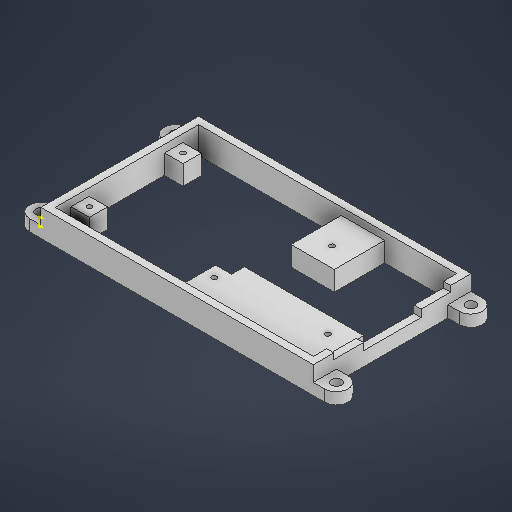
# Autodesk Inventor part: lock2
Saved by Autodesk Inventor 2026 (Build 300175050, 175E)
## iProperties
Created: 2025-07-25
Part Number: lock2
Material: Generic
Document SubType Name: Modeling
Designer: User
Density: 1 g/cm^3
Appearance: Default
Author: User
Autodesk Inventor part; units mm, degrees
ref_plane "YZ Plane" through (0, 0, 0) normal (1, 0, 0) x (0, 1, 0)
ref_plane "XZ Plane" through (0, 0, 0) normal (0, 1, 0) x (-1, 0, 0)
ref_plane "XY Plane" through (0, 0, 0) normal (0, 0, 1) x (1, 0, 0)
sketch "Sketch1" plane through (0, 0, 0) normal (0, 1, 0) x (-1, 0, 0)
  line L0 (0, 0) -> (-94.5, 0)
  line L1 (-94.5, 0) -> (-94.5, -54.7)
  line L2 (-94.5, -54.7) -> (0, -54.7)
  line L3 (0, -54.7) -> (0, 0)
  dimension "d0" = 94.5
  dimension "d1" = 54.7
  constraints: 8 end point, 2 parallel, 1 horizontal, 1 perpendicular
  measures "d0" distance of L2.end L1.end
  measures "d1" distance of L1.end L0.end
extrude "Extrusion1" add sketch "Sketch1" along normal blind 9.3
sketch "Sketch2" plane through (0, 9.3, 0) normal (0, 1, 0) x (1, 0, 0)
  line L0 (2.5, 2.5) -> (92, 2.5)
  line L1 (92, 2.5) -> (92, 52.2)
  line L2 (92, 52.2) -> (2.5, 52.2)
  line L3 (2.5, 52.2) -> (2.5, 2.5)
  line L4 (0, 0) -> (94.5, 0) projected
  line L5 (0, 54.7) -> (0, 0) projected
  dimension "d4" = 89.5
  dimension "d5" = 49.7
  dimension "d6" = 2.5
  dimension "d7" = 2.5
  constraints: 8 end point, 2 parallel, 1 horizontal, 1 perpendicular
  measures "d4" distance of L2.end L1.end
  measures "d5" distance of L1.end L0.end
  measures "d6" distance between parallel lines of L4 L0
  measures "d7" distance between parallel lines of L5 L3
extrude "Extrusion2" cut sketch "Sketch2" against normal blind 2.5
sketch "Sketch3" plane through (0, 6.8, 0) normal (0, 1, 0) x (1, 0, 0)
  point P0 (0, 0)
sketch "Sketch4" plane through (0, 6.8, 0) normal (0, 1, 0) x (1, 0, 0)
  line L0 (2.6094, 40.3) -> (9.0094, 40.3)
  line L1 (9.0094, 40.3) -> (9.0094, 46.6)
  line L2 (9.0094, 46.6) -> (2.6094, 46.6)
  line L3 (2.6094, 46.6) -> (2.6094, 40.3)
  line L4 (2.5, 52.2) -> (92, 52.2) projected
  line L5 (2.5, 2.5) -> (2.5, 52.2) projected
  line L6 (2.5, 7.905) -> (8.9, 7.905)
  line L7 (8.9, 7.905) -> (8.9, 14.205)
  line L8 (8.9, 14.205) -> (2.5, 14.205)
  line L9 (2.5, 14.205) -> (2.5, 7.905)
  line L10 (92, 2.5) -> (2.5, 2.5) projected
  line L11 (45.1276, 2.5) -> (95.6526, 2.5)
  line L12 (95.6526, 2.5) -> (95.6526, 19.973)
  line L13 (95.6526, 19.973) -> (45.1276, 19.973)
  line L14 (45.1276, 19.973) -> (45.1276, 2.5)
  line L15 (52.018, 52.2) -> (67.018, 52.2)
  line L16 (67.018, 52.2) -> (67.018, 34.727)
  line L17 (67.018, 34.727) -> (52.018, 34.727)
  line L18 (52.018, 34.727) -> (52.018, 52.2)
  line L19 (92, 52.2) -> (92, 2.5) projected
  point P0 (0, 0)
  point P1 (5.8094, 46.6)
  point P2 (5.7, 7.905)
  point P3 (67.018, 43.4635)
  point P4 (92, 19.973)
  point P5 (2.5, 14.205)
  dimension "d10" = 6.4
  dimension "d11" = 6.3
  dimension "d12" = 5.6
  dimension "d13" = 6.4
  dimension "d14" = 6.3
  dimension "d15" = 5.405
  dimension "d16" = 50.525
  dimension "d17" = 17.473
  dimension "d18" = 15
  dimension "d19" = 17.473
  dimension "d20" = 24.982
  constraints: 32 end point, 8 parallel, 4 horizontal, 4 perpendicular, 3 midpoint, 3 point on line
  measures "d10" distance of L2.end L1.end
  measures "d11" distance of L1.end L0.end
  measures "d12" distance from line of L4 point (5.809, 46.6)
  measures "d13" distance of L8.end L7.end
  measures "d14" distance of L7.end L6.end
  measures "d15" distance from line of point (5.7, 7.905) L10
  measures "d16" distance of L13.end L12.end
  measures "d17" distance of L12.end L11.end
  measures "d18" distance of L16.end L17.end
  measures "d19" distance of L15.end L16.end
  measures "d20" distance from line of L19 point (67.018, 43.464)
extrude "Extrusion3" cut sketch "Sketch4" against normal blind 10 contours L4 L18 L17 L16 L19 L13 L14 L10 L5 L6 L7 L8
sketch "Sketch5" plane through (0, 6.8, 0) normal (0, 1, 0) x (1, 0, 0)
  line L0 (45.1276, 2.5) -> (45.1276, 19.973) projected
  line L1 (45.1276, 19.973) -> (50.6276, 19.973)
  line L2 (50.6276, 19.973) -> (50.6276, 15.473)
  line L3 (50.6276, 15.473) -> (45.1276, 15.473)
  line L4 (45.1276, 15.473) -> (45.1276, 19.973)
  point P0 (0, 0)
  dimension "d23" = 5.5
  dimension "d24" = 4.5
  constraints: 8 end point, 2 parallel, 1 horizontal, 1 perpendicular
  measures "d23" distance of L2.end L3.end
  measures "d24" distance of L1.end L2.end
extrude "Extrusion4" cut sketch "Sketch5" against normal blind 10
sketch "Sketch6" plane through (0, 9.3, 0) normal (0, 1, 0) x (1, 0, 0)
  line L0 (92, 19.973) -> (92, 2.5) projected
  line L1 (94.5, 0) -> (94.5, 54.7) projected
  line L2 (92, 7.1) -> (94.5, 7.1)
  line L3 (94.5, 7.1) -> (94.5, 47.6)
  line L4 (94.5, 47.6) -> (92, 47.6)
  line L5 (92, 47.6) -> (92, 7.1)
  line L6 (94.5, 54.7) -> (0, 54.7) projected
  point P0 (0, 0)
  point P1 (93.25, 47.6)
  dimension "d27" = 40.5
  dimension "d28" = 7.1
  constraints: 8 end point, 2 parallel, 2 point on line, 1 horizontal, 1 midpoint, 1 perpendicular
  measures "d27" distance of L3.end L2.end
  measures "d28" distance from line of L6 point (93.25, 47.6)
extrude "Extrusion5" cut sketch "Sketch6" against normal blind 2
sketch "Sketch7" plane through (0, 7.3, 0) normal (0, 1, 0) x (1, 0, 0)
  line L0 (92, 19.973) -> (92, 2.5) projected
  line L1 (94.5, 0) -> (94.5, 54.7) projected
  line L2 (92, 17.35) -> (94.5, 17.35)
  line L3 (94.5, 17.35) -> (94.5, 37.35)
  line L4 (94.5, 37.35) -> (92, 37.35)
  line L5 (92, 37.35) -> (92, 17.35)
  line L6 (92, 47.6) -> (94.5, 47.6) projected
  point P0 (0, 0)
  point P1 (93.25, 47.6)
  point P2 (93.25, 37.35)
  dimension "d31" = 20
  dimension "d32" = 10.25
  constraints: 8 end point, 2 midpoint, 2 parallel, 2 point on line, 1 horizontal, 1 perpendicular
  measures "d31" distance of L3.end L2.end
  measures "d32" distance of point (93.25, 47.6) point (93.25, 37.35)
extrude "Extrusion6" cut sketch "Sketch7" against normal blind 2.5
sketch "Sketch8" plane through (0, 0, -54.7) normal (-1, 0, 0) x (0, 0, 1)
  line L0 (54.7, 0) -> (46.7, 0)
  line L1 (46.7, 0) -> (46.7, 4)
  line L2 (46.7, 4) -> (54.7, 4)
  line L3 (54.7, 4) -> (54.7, 0)
  line L4 (0, 0) -> (0, 9.3) projected
  line L5 (0, 0) -> (8, 0)
  line L6 (8, 0) -> (8, 4)
  line L7 (8, 4) -> (0, 4)
  line L8 (0, 4) -> (0, 0)
  point P0 (0, 4)
  point P1 (4, 0)
  point P2 (4, 4)
  dimension "d35" = 8
  dimension "d36" = 4
  dimension "d37" = 8
  dimension "d47" = 4
  constraints: 16 end point, 4 parallel, 2 horizontal, 2 midpoint, 2 perpendicular, 1 point on line
  measures "d35" distance of L1.end L2.end
  measures "d36" distance of L0.end L1.end
  measures "d37" distance of L7.end L6.end
  measures "d47" distance of point (4, 0) point (4, 4)
extrude "Extrusion7" add sketch "Sketch8" along normal blind 8
sketch "Sketch9" plane through (94.5, 0, 0) normal (1, 0, 0) x (0, 0, -1)
  line L0 (0, 0) -> (8, 0)
  line L1 (8, 0) -> (8, 4)
  line L2 (8, 4) -> (0, 4)
  line L3 (0, 4) -> (0, 0)
  line L4 (54.6278, 0) -> (46.6278, 0)
  line L5 (46.6278, 0) -> (46.6278, 4)
  line L6 (46.6278, 4) -> (54.6278, 4)
  line L7 (54.6278, 4) -> (54.6278, 0)
  dimension "d40" = 8
  dimension "d41" = 4
  dimension "d42" = 8
  dimension "d43" = 4
  constraints: 16 end point, 4 parallel, 2 horizontal, 2 perpendicular, 1 point on line
  measures "d40" distance of L2.end L1.end
  measures "d41" distance of L1.end L0.end
  measures "d42" distance of L5.end L6.end
  measures "d43" distance of L4.end L5.end
extrude "Extrusion8" add sketch "Sketch9" along normal blind 8
fillet "Fillet1" radius 4 8 edges at (102.5, 2, 0) (102.5, 2, -8) (102.5, 2, -46.6278) (102.5, 2, -54.6278) (-8, 2, 0) (-8, 2, -8) (-8, 2, -46.7) (-8, 2, -54.7)
sketch "Sketch10" plane through (94.5, 4, -46.6278) normal (0, 1, 0) x (1, 0, 0)
  point P0 (-94.5, -46.6278)
sketch "Sketch11" plane through (0, 4, 0) normal (0, 1, 0) x (1, 0, 0)
  circle A0 centre (-4, 4) radius 1.75
  line L0 (0, 8) -> (-4, 8) projected
  line L1 (0, 54.7) -> (0, 0) projected
  dimension "d48" = 3.5
  dimension "d49" = 4
  dimension "d50" = 4
  constraints: 1 centre point
  measures "d48" diameter of A0
  measures "d49" distance from line of L0 A0.centre
  measures "d50" distance from line of L1 A0.centre
extrude "Extrusion9" cut sketch "Sketch11" against normal blind 8
sketch "Sketch12" plane through (0, 4, -46.7) normal (0, 1, 0) x (1, 0, 0)
  circle A0 centre (-4, 4) radius 1.75
  line L0 (0, 8) -> (0, -46.7) projected
  line L1 (0, 8) -> (-4, 8) projected
  dimension "d53" = 3.5
  dimension "d54" = 4
  dimension "d55" = 4
  constraints: 1 centre point
  measures "d53" diameter of A0
  measures "d54" distance from line of L0 A0.centre
  measures "d55" distance from line of L1 A0.centre
extrude "Extrusion10" cut sketch "Sketch12" against normal blind 8
sketch "Sketch13" plane through (94.5, 4, 0) normal (0, 1, 0) x (1, 0, 0)
  circle A0 centre (4, 4) radius 1.75
  circle A1 centre (4, 50.6278) radius 1.75
  line L0 (0, 8) -> (4, 8) projected
  line L1 (0, 0) -> (0, 7.1) projected
  line L2 (0, 54.6278) -> (4, 54.6278) projected
  line L3 (0, 47.6) -> (0, 54.7) projected
  point P0 (-94.5, 0)
  point P1 (0, 3.55)
  dimension "d58" = 3.5
  dimension "d59" = 3.5
  dimension "d60" = 4
  dimension "d61" = 4
  dimension "d62" = 4
  dimension "d63" = 4
  constraints: 2 centre point, 1 midpoint
  measures "d58" diameter of A0
  measures "d59" diameter of A1
  measures "d60" distance from line of L0 A0.centre
  measures "d61" horizontal distance of point (0, 3.55) A0.centre
  measures "d62" distance from line of L2 A1.centre
  measures "d63" distance from line of L3 A1.centre
extrude "Extrusion11" cut sketch "Sketch13" against normal blind 8
sketch "Sketch14" plane through (0, 6.8, 0) normal (0, 1, 0) x (1, 0, 0)
  circle A0 centre (5.7, 11.105) radius 0.875
  circle A1 centre (5.8094, 43.5) radius 0.875
  line L0 (8.9, 7.905) -> (8.9, 14.205) projected
  line L1 (2.5, 7.905) -> (8.9, 7.905) projected
  line L2 (9.0094, 40.3) -> (9.0094, 46.6) projected
  line L3 (2.6094, 40.3) -> (9.0094, 40.3) projected
  circle A2 centre (57.5534, 40.3) radius 0.875
  line L4 (52.018, 34.727) -> (67.018, 34.727) projected
  point P0 (0, 0)
  point P1 (5.7, 7.905)
  point P2 (9.0094, 43.45)
  point P3 (5.8094, 40.3)
  point P4 (59.518, 34.727)
  dimension "d66" = 1.75
  dimension "d67" = 1.75
  dimension "d68" = 3.2
  dimension "d69" = 3.2
  dimension "d70" = 3.2
  dimension "d71" = 3.2
  dimension "d72" = 1.75
  dimension "d73" = 5.573
  constraints: 4 midpoint, 3 centre point
  measures "d66" diameter of A0
  measures "d67" diameter of A1
  measures "d68" distance from line of L0 A0.centre
  measures "d69" distance of point (5.7, 7.905) A0.centre
  measures "d70" horizontal distance of point (9.009, 43.45) A1.centre
  measures "d71" distance of point (5.809, 40.3) A1.centre
  measures "d72" diameter of A2
  measures "d73" vertical distance of point (59.518, 34.727) A2.centre
extrude "Extrusion12" cut sketch "Sketch14" against normal blind 2.5 contours A0 | A1
sketch "Sketch15" plane through (0, 6.8, 0) normal (0, 1, 0) x (1, 0, 0)
  circle A0 centre (59.578, 41.427) radius 0.875
  line L0 (52.018, 52.2) -> (52.018, 34.727) projected
  line L1 (52.018, 34.727) -> (67.018, 34.727) projected
  point P0 (0, 0)
  point P1 (59.518, 34.727)
  dimension "d76" = 1.75
  dimension "d77" = 7.56
  dimension "d78" = 6.7
  constraints: 1 centre point, 1 midpoint
  measures "d76" diameter of A0
  measures "d77" distance from line of L0 A0.centre
  measures "d78" vertical distance of point (59.518, 34.727) A0.centre
extrude "Extrusion13" cut sketch "Sketch15" against normal blind 2.5
sketch "Sketch16" plane through (0, 6.8, 0) normal (0, 1, 0) x (1, 0, 0)
  circle A0 centre (48.6276, 11.473) radius 0.875
  circle A1 centre (85.359, 14.173) radius 0.875
  line L0 (50.6276, 15.473) -> (45.1276, 15.473) projected
  line L1 (45.1276, 15.473) -> (45.1276, 2.5) projected
  line L2 (92, 7.1) -> (92, 17.35) projected
  line L3 (92, 19.973) -> (50.6276, 19.973) projected
  point P0 (0, 0)
  point P1 (47.8776, 15.473)
  dimension "d81" = 1.75
  dimension "d82" = 1.75
  dimension "d83" = 4
  dimension "d84" = 3.5
  dimension "d85" = 6.641
  dimension "d86" = 5.8
  constraints: 2 centre point, 1 midpoint
  measures "d81" diameter of A0
  measures "d82" diameter of A1
  measures "d83" vertical distance of point (47.878, 15.473) A0.centre
  measures "d84" distance from line of L1 A0.centre
  measures "d85" distance from line of L2 A1.centre
  measures "d86" distance from line of L3 A1.centre
extrude "Extrusion14" cut sketch "Sketch16" against normal blind 2.5
body "Solid1"
